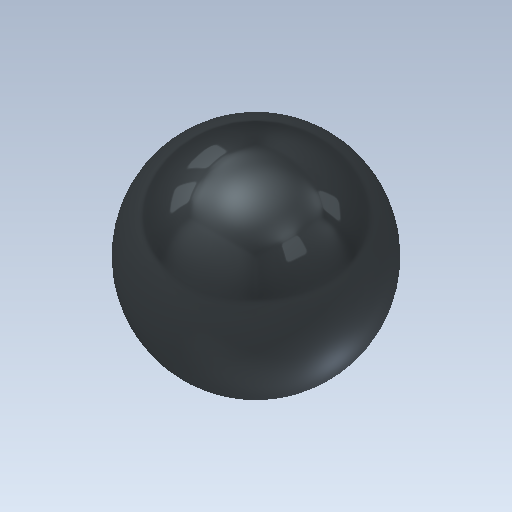
# Autodesk Inventor part: 6900ZZ Ball
Saved by Autodesk Inventor 2021 (Build 250183000, 183)
## iProperties
Category: PARTsolutions
Company: NTN
Created: 2019-07-31
Part Number: 6900ZZ Ball
Material: 鉄、鋳鉄
Catalog Web Link: www.cadenas.de
Description: Open type ball-Deep Groove Ball Bearings
Vendor: NTN
Document SubType Name: Modeling
Designer: psadmin
Manufacturer: NTN
Mass: 0.166079 g
Surface Area: 0.393692 cm^2
Volume: 0.0232278 cm^3
Density: 7.15 g/cm^3
Appearance: 鉄 灰色
PSOL_IDENT_0: {$CADENAS_DATA\23d-libs\ntn\ball_roller_bearings\deep_groove_bb\deep_groove_bb\6_types\dgbb_ball.prj
PSOL_IDENT_1: },172 {VTYP=3D},{NB=6900ZZ Ball},{LINA=6900ZZ Ball},{NN=Open type ball},{DATE=29.01.2019 23:03:43},{
PSOL_IDENT_2: GEOMDATE=14.01.2008 00:00:00},{VERSION=},{LINEID=2800},{WBVAR=},{WBNUMERIC=}  {NB=6900ZZ Ball},{LINA=
PSOL_IDENT_3: 6900ZZ Ball},{KT=DUMMY},{IDNR=},{SD=10},{D=22},{B=6},{R=0.3},{ORDER1=6900},{ORDER=6900ZZ},{CR=2.70},
PSOL_IDENT_4: {COR=1.27},{CRF=275},{CORF=129},{LSG=30000},{LSO=36000},{MASS=0.01},{RNS=0.3},{LLH=0},{LLU=21000},{S
PSOL_IDENT_5: T=ZZ},{NCST=LLB},{LTST=0},{CST=LLU},{SRG=N},{SR=NR},{D1=20.80},{A=1.05},{BA=0.80},{R0=0.20},{D2=24.8
PSOL_IDENT_6: },{F=0.70},{DA1=12},{DA2=13},{DA=20},{DX=25.5},{CY=1.5},{CZ=0.7},{RAS=0.3},{RNAS=0.3},{VERS=2},{X=6}
NN: Open type ball
NT: Deep Groove Ball Bearings
NB: 6900ZZ Ball
NBSYN: $ORDER. Ball
LINA: 6900ZZ Ball
SD: 10
D: 22
B: 6
R: 0.3
ORDER1: 6900
CR: 2.70
COR: 1.27
CRF: 275
CORF: 129
LSG: 30000
LSO: 36000
MASS: 0.01
RNS: 0.3
LLH: 0
LLU: 21000
ST: ZZ
NCST: LLB
LTST: 0
CST: LLU
SRG: N
SR: NR
D1: 20.8
A: 1.05
BA: 0.8
R0: 0.2
D2: 24.8
F: 0.7
DA1: 12
DA2: 13
DA: 20
DX: 25.5
CY: 1.5
CZ: 0.7
RAS: 0.3
RNAS: 0.3
VERS: 2
SUPPLIER: NTN
ARTICLENO: 6900ZZ Ball
BOMINFO: 6900ZZ Ball
CREATOR: CADENAS GmbH
Title: 6900ZZ Ball
Author: Cadenas PARTsolutions
Comments: Deep Groove Ball Bearings
Autodesk Inventor part; units mm, degrees
sketch "Sketch_1" plane through (0, 0, 0) normal (0, 0, 1) x (1, 0, 0)
  line L0 (1.77, 0) -> (-1.77, 0)
  arc A0 (1.77, 0) -> (-1.77, 0) centre (0, 0) ccw
  line L1 (1.77, 0) -> (-1.77, 0)
  constraints: 4 end point, 2 point on circle, 1 centre point
revolve "Revolution1" add sketch "Sketch_1" angle 360 about axis through (1.77, 0, 0) along (1, 0, 0)
ref_plane "dgbb_ball_XY" through (0, 0, 0) normal (1, 0, 0) x (0, 0, -1)
ref_plane "dgbb_ball_YZ" through (0, 0, 0) normal (0, 0, -1) x (0, 1, 0)
ref_plane "dgbb_ball_ZX" through (0, 0, 0) normal (0, 1, 0) x (1, 0, 0)
body "Solid1"
